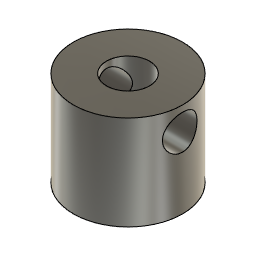
NeckConnector3 v4 (Autodesk Fusion 360 design; units mm, degrees)
Autodesk Fusion 360 part; units mm, degrees
sketch "ServoSideBase" plane through (0, 0, 0) normal (0, 0, 1) x (1, 0, 0) in component "ServoSide"
  circle A0 centre (0, 0) radius 10.4
  circle A1 centre (0, 0) radius 4.1
  dimension "d3" = 20.8
  dimension "d4" = 8.2
  constraint coincident A0.centre A1.centre
  constraint concentric A0 A1
  measures "d3" diameter of A0
  measures "d4" diameter of A1
extrude "ExtrudeServoSideBase" add sketch "ServoSideBase" along normal blind 18 in component "ServoSide"
sketch "ServoScrews" plane through (0, 0, 0) normal (0, 0, -1) x (1, 0, 0) in component "ServoSide"
  circle A0 centre (0, 0) radius 4.1
  circle A1 centre (0, 0) radius 10.4
  line L0 (0, 10.4) -> (0, -10.4) construction
  line L1 (-10.4, 0) -> (10.4, 0) construction
  circle A2 centre (0, 7.75) radius 0.8
  circle A3 centre (-7.75, 0) radius 0.8
  circle A4 centre (0, -7.75) radius 0.8
  circle A5 centre (7.75, 0) radius 0.8
  point P0 (0, 7.75)
  dimension "d7" = 7.75
  dimension "d8" = 1.6
  dimension "d10" = 360
  constraint coincident A1 L0.start
  constraint coincident A1 L0.end
  constraint vertical L0
  constraint coincident A0.centre L0
  constraint coincident A1 L1.start
  constraint coincident A1 L1.end
  constraint horizontal L1
  constraint coincident A0.centre L1
  constraint coincident L0 P0
  constraint coincident P0 A2.centre
  measures "d7" distance of A0.centre A2.centre
  measures "d8" diameter of A2
extrude "CutServoScrewHoles" cut sketch "ServoScrews" against normal blind 4 contours A2 | A3 | A4 | A5 in component "ServoSide"
sketch "LargeScrewHole" plane through (0, 0, 0) normal (1, 0, 0) x (0, 1, 0) in component "ServoSide"
  line L0 (0, 18) -> (0, 0) construction
  circle A0 centre (0, 13.5) radius 3.3
  point P0 (0, 18)
  dimension "d41" = 6.6
  dimension "d42" = 4.5
  constraint coincident P0 L0.start
  constraint coincident L0.end origin
  constraint coincident L0 A0.centre
  measures "d41" diameter of A0
  measures "d42" distance of P0 A0.centre
extrude "ExtrudeScrewHole" cut sketch "LargeScrewHole" along normal through all and the other way through all in component "ServoSide"
component "ServoSide" placed x (1, 0, 0) y (0, 1, 0) z (0, 0, 1) at (0, 0, 0)
equation "outside_diam = 20.8 mm"
equation "inside_diam = 8.2 mm"
equation "d3 = outside_diam"
equation "d4 = inside_diam"
equation "d5 = servoside_height"
equation "servoside_height = 18 mm"
equation "slop = 0.1 mm"
equation "neckside_height = 16 mm"
equation "sm_screw_diam = 3.9 mm"
equation "lg_screw_diam = 6.4 mm"
named bodies: "ServoSide"
